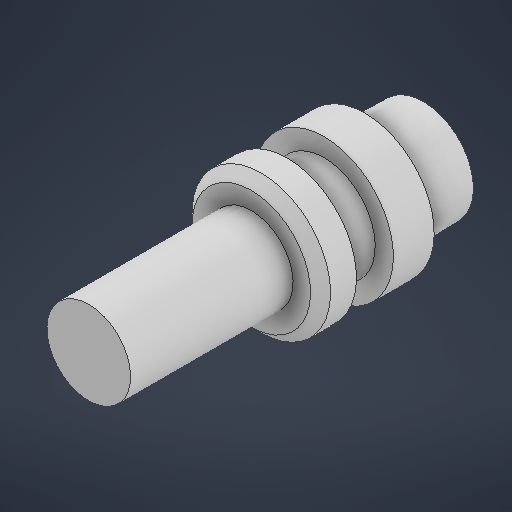
# Autodesk Inventor part: simple_shaft
Saved by Autodesk Inventor 2026 (Build 300175050, 175E)
## iProperties
Created: 2025-09-17
Part Number: simple_shaft
Material: Generic
Document SubType Name: Modeling
Designer: Administrator
Density: 1 g/cm^3
Appearance: Default
Author: Administrator
Autodesk Inventor part; units mm, degrees
ref_plane "YZ Plane" through (0, 0, 0) normal (1, 0, 0) x (0, 1, 0)
ref_plane "XZ Plane" through (0, 0, 0) normal (0, 1, 0) x (-1, 0, 0)
ref_plane "XY Plane" through (0, 0, 0) normal (0, 0, 1) x (1, 0, 0)
sketch "Sketch1" plane through (0, 0, 0) normal (1, 0, 0) x (0, 1, 0)
  line L0 (0, 17.706) -> (3.1851, 17.706)
  line L1 (3.1851, 17.706) -> (3.1851, 5.3262)
  line L2 (3.1851, 5.3262) -> (5.2739, 5.3262)
  line L3 (5.2739, 5.3262) -> (5.2739, 2.5911)
  line L4 (5.2739, 2.5911) -> (3.8979, 2.5911)
  line L5 (3.8979, 2.5911) -> (3.8979, -0.2159)
  line L6 (3.8979, -0.2159) -> (5.2809, -0.2159)
  line L7 (5.2809, -0.2159) -> (5.2809, -3.3244)
  line L8 (5.2809, -3.3244) -> (3.8979, -3.3008)
  line L9 (3.8979, -3.3008) -> (3.8214, -7.7742)
  line L10 (3.8214, -7.7742) -> (0, -7.7742)
  line L11 (0, -7.7742) -> (0, 17.706)
  point P0 (0, 0)
  constraints: 24 end point, 9 perpendicular, 1 horizontal, 1 parallel, 1 point on line
revolve "Revolution1" add sketch "Sketch1" angle 360 about axis through (0, 0, -7.7742) along (0, 0, 1)
chamfer "Chamfer1" distance 0.762 angle 45 1 edges at (0, -5.2739, 5.3262)
body "Solid1"
